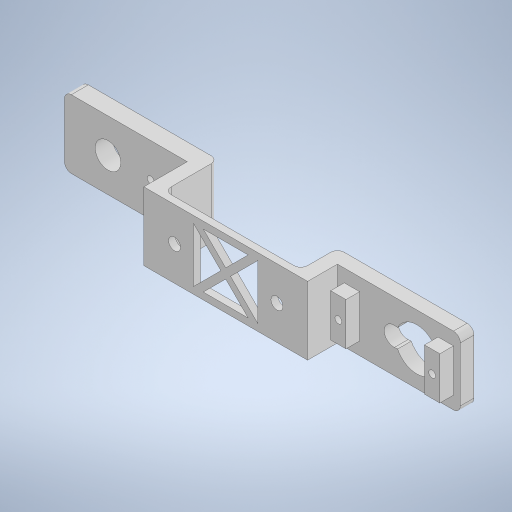
# Autodesk Inventor part: joint2_servo
Saved by Autodesk Inventor 2023 (Build 270158000, 158)
## iProperties
Created: 2023-04-29
Part Number: joint2_servo
Material: 一般
Document SubType Name: Modeling
Designer: taka2
Density: 1 g/cm^3
Appearance: 既定
Author: taka2
Autodesk Inventor part; units mm, degrees
ref_plane "YZ Plane" through (0, 0, 0) normal (1, 0, 0) x (0, 1, 0)
ref_plane "XZ Plane" through (0, 0, 0) normal (0, 1, 0) x (-1, 0, 0)
ref_plane "XY Plane" through (0, 0, 0) normal (0, 0, 1) x (1, 0, 0)
sketch "スケッチ1" plane through (0, 0, 0) normal (0, 0, 1) x (1, 0, 0)
  line L0 (-12.75, -10) -> (27.25, -10)
  line L1 (27.25, -10) -> (27.25, 10)
  line L2 (27.25, 10) -> (-12.75, 10)
  line L3 (-12.75, 10) -> (-12.75, -10)
  line L4 (23.25, 10) -> (23.25, -10)
  line L5 (-37.0617, 0) -> (56.2147, 0)
  point P0 (27.25, 0)
  dimension "d9" = 20
  dimension "d30" = 4
  dimension "d94" = 40
  constraints: 12 end point, 3 point on line, 2 horizontal, 2 parallel, 2 perpendicular, 1 midpoint
  measures "d9" distance of L2.end L0.start
  measures "d30" distance between parallel lines of L1 L4
  measures "d94" distance of L1.end L2.end
extrude "押し出し1" add sketch "スケッチ1" along normal blind 4 and the other way blind 1
extrude "押し出し4" add sketch "スケッチ1" along normal blind 16.75 contours L4 L5 L1 L0 | L4 L2 L1 L5
sketch "スケッチ2" plane through (0, 0, 16.75) normal (0, 0, 1) x (1, 0, 0)
  line L0 (23.25, -10) -> (23.25, 10) projected
  line L1 (23.25, 0) -> (71.25, 0)
  line L2 (23.25, 10) -> (71.25, 10)
  line L3 (71.25, 10) -> (71.25, -10)
  line L4 (71.25, -10) -> (23.25, -10)
  line L5 (37.8358, 8) -> (37.8358, -8)
  line L6 (37.8358, -8) -> (53.8358, -8)
  line L7 (53.8358, -8) -> (37.8358, 8)
  circle A0 centre (32.25, 0) radius 1.75
  circle A1 centre (32.25, 0) radius 3
  line L8 (27.25, -10) -> (27.25, 10) projected
  line L9 (67.25, 10) -> (67.25, -10)
  line L10 (56.6642, 8) -> (56.6642, -8)
  line L11 (47.25, 10) -> (47.25, -10)
  circle A2 centre (62.25, 0) radius 1.75
  circle A3 centre (62.25, 0) radius 3
  line L12 (56.6642, 8) -> (40.6642, 8)
  line L13 (40.6642, 8) -> (56.6642, -8)
  line L14 (56.6642, 8) -> (40.6642, -8)
  line L15 (37.8358, -8) -> (53.8358, 8)
  point P0 (0, 0)
  point P1 (47.25, -8)
  point P2 (45.8358, 0)
  point P3 (47.25, 0)
  point P4 (47.25, 1.4142)
  point P5 (48.6642, 0)
  point P6 (47.25, -1.4142)
  point P7 (45.8358, 0)
  point P8 (47.25, -1.4142)
  point P9 (47.25, 1.4142)
  point P10 (48.6642, 0)
  dimension "d33" = 3.5
  dimension "d34" = 6
  dimension "d37" = 16
  dimension "d43" = 4
  dimension "d63" = 48
  dimension "d64" = 30
  dimension "d65" = 2
  dimension "d100" = 2
  constraints: 28 end point, 7 point on line, 4 centre point, 4 horizontal, 4 midpoint, 4 symmetric about line, 3 perpendicular, 2 coincident, 2 equal length, 2 parallel, 2 vertical, 3 other
  measures "d33" diameter of A0
  measures "d34" diameter of A1
  measures "d37" distance of L5.start L5.end
  measures "d43" distance between parallel lines of L3 L9
  measures "d63" distance between parallel lines of L3 L0
  measures "d64" distance of A2.centre A0.centre
  measures "d65" distance between parallel lines of L7 L13
  measures "d100" distance between parallel lines of L14 L15
extrude "押し出し5" add sketch "スケッチ2" against normal blind 2 contours L8 L1 A1 L5 L6 L11 L4 | L8 L2 L11 L12 L13 L15 L7 L5 L1 A1 | L11 L6 L7 L14 L13 L10 L1 A3 L9 L4 | A1 L1 A0 | L1 A0 A1 | L2 L9 L1 A3 L10 L12 L11 | L6 L15 L7 L14 | L7 L1 L11 | L11 L1 L14 | A3 L1 A2 | L1 A2 A3 | L15 L11 L1 | L11 L13 L1 | L13 L15 L12 L14
extrude "押し出し6" add sketch "スケッチ2" against normal blind 12.75 contours L9 L1 L3 L4 | L9 L2 L3 L1
sketch "スケッチ5" plane through (0, 0, 4) normal (0, 0, -1) x (-1, 0, 0)
  line L0 (-67.25, -10) -> (-67.25, 10)
  line L1 (-67.25, -10) -> (-107.25, -10)
  line L2 (-107.25, -10) -> (-107.25, 10)
  line L3 (-107.25, 10) -> (-67.25, 10)
  line L4 (-105.25, -6.25) -> (-73.25, -6.25)
  line L5 (-73.25, -6.25) -> (-73.25, 6.25)
  line L6 (-73.25, 6.25) -> (-105.25, 6.25)
  line L7 (-105.25, 6.25) -> (-105.25, -6.25)
  line L8 (-77.75, -6.25) -> (-77.75, 6.25)
  line L9 (-100.75, -6.25) -> (-100.75, 6.25)
  line L10 (-71.25, 10) -> (-71.25, -10)
  line L11 (-71.25, 0) -> (-107.25, 0)
  arc A0 (-88.8773, 2.7291) -> (-88.8773, -2.7291) centre (-94.5, 0) ccw
  arc A1 (-87.9419, -2.7934) -> (-87.9419, 2.7934) centre (-87.75, 0) ccw
  line L12 (-87.9419, -2.7934) -> (-88.8773, -2.7291)
  line L13 (-87.9419, 2.7934) -> (-88.8773, 2.7291)
  circle A2 centre (-103, 0) radius 1
  circle A3 centre (-75.5, 0) radius 1
  point P0 (0, 0)
  point P1 (0, 0)
  point P2 (-94.5, -6.25)
  point P3 (-94.5, 6.25)
  point P4 (-100.75, 0)
  dimension "d76" = 2
  dimension "d77" = 12.5
  dimension "d78" = 4.5
  dimension "d79" = 4.5
  dimension "d80" = 2.25
  dimension "d81" = 2.25
  dimension "d82" = 23
  dimension "d83" = 13
  dimension "d84" = 2.8
  dimension "d85" = 2
  dimension "d86" = 2
  constraints: 29 end point, 11 point on line, 4 centre point, 4 perpendicular, 4 point on circle, 3 tangent, 2 midpoint, 2 parallel, 2 vertical, 1 equal radius, 2 other
  measures "d76" diameter of A2
  measures "d77" distance of L7.start L7.end
  measures "d78" distance of L9.end L7.start
  measures "d79" distance of L8.end L5.end
  measures "d80" distance from line of L7 A2.centre
  measures "d81" distance from line of L5 A3.centre
  measures "d82" distance of L9.end L8.end
  measures "d83" distance from line of A1.centre L9
  measures "d84" radius of A1
  measures "d85" distance between parallel lines of L5 L10
  measures "d86" distance between parallel lines of L2 L7
extrude "押し出し11" add sketch "スケッチ5" against normal blind 4 contours L1 L2 L11 L7 L4 L5 L10 | L10 L11 L5 L6 L7 L2 L3 | L4 A0 L12 A1 L11 L8 | L8 L11 A1 L13 A0 L6 | L6 A0 L9 | L9 A0 L4
extrude "押し出し13" add sketch "スケッチ5" against normal blind 8 contours L11 A3 L8 L6 L5 | L5 L4 L8 L11 A3 | L11 A2 L9 L4 L7 | L7 L6 L9 L11 A2
sketch "スケッチ4" plane through (0, 0, -1) normal (0, 0, -1) x (-1, 0, 0)
  circle A0 centre (0, 0) radius 3.75
  arc A1 (-14.3614, 2.0436) -> (-14.3614, -2.0436) centre (-14.2, 0) ccw
  line L0 (12.75, 10) -> (12.75, -10) projected
  line L1 (12.75, 0) -> (-27.25, 0)
  line L2 (-27.25, 10) -> (-27.25, -10) projected
  line L3 (-14.3614, 2.0436) -> (-2.25, 3)
  line L4 (-14.3614, -2.0436) -> (-2.25, -3)
  circle A2 centre (-12.5, 0) radius 1
  dimension "d66" = 7.5
  dimension "d67" = 14.2
  dimension "d68" = 6
  dimension "d69" = 2.05
  dimension "d70" = 2
  dimension "d71" = 12.5
  constraints: 6 end point, 4 point on circle, 3 centre point, 2 midpoint, 2 tangent, 1 coincident, 1 point on line, 1 other
  measures "d66" diameter of A0
  measures "d67" distance of point (0, 0) A1.centre
  measures "d68" distance of L4.end L3.end
  measures "d69" radius of A1
  measures "d70" diameter of A2
  measures "d71" distance of A2.centre point (0, 0)
extrude "押し出し9" cut sketch "スケッチ4" against normal through all contours L1 A0 | A0 L1 | A2 L1 | L1 A2
extrude "押し出し10" cut sketch "スケッチ4" against normal blind 1.5 contours A0 L1 A2 A1 L3 | L4 A1 L1 A2 A0
fillet "フィレット1" radius 2 4 edges at (-12.75, 10, 1.5) (107.25, 10, 6) (107.25, -10, 6) (-12.75, -10, 1.5)
fillet "フィレット2" radius 2 4 edges at (27.25, 0, -1) (67.25, 0, 14.75) (67.25, 0, 4) (27.25, 0, 14.75)
